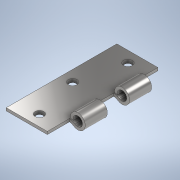
# Autodesk Inventor part: Hinge1
Saved by Autodesk Inventor 2021 (Build 250183000, 183)
## iProperties
Created: 2021-07-31
Part Number: Hinge1
Material: Stainless Steel
Document SubType Name: Modeling
Designer: Shammy Haider
Density: 8 g/cm^3
Appearance: Semi-Polished
Author: Shammy Haider
Autodesk Inventor part; units mm, degrees
ref_plane "YZ Plane" through (0, 0, 0) normal (1, 0, 0) x (0, 1, 0)
ref_plane "XZ Plane" through (0, 0, 0) normal (0, 1, 0) x (-1, 0, 0)
ref_plane "XY Plane" through (0, 0, 0) normal (0, 0, 1) x (1, 0, 0)
sketch "Sketch1" plane through (0, 0, 0) normal (0, 0, 1) x (1, 0, 0)
  line L0 (-44.6809, 2.5) -> (-7.5647, 2.5)
  line L1 (-44.6809, 0) -> (-44.6809, 2.5)
  line L2 (0, 0) -> (0, 19.2246)
  arc A0 (-3.8253, -1.3563) -> (-6.7141, 3.5099) centre (0, 4.2052) ccw
  arc A1 (-2.5687, 0.8193) -> (-4.0285, 2.8511) centre (0, 4.2052) ccw
  arc A2 (-2.5687, 0.8193) -> (-7.5647, 2.5) centre (-7.5647, -5.7659) ccw
  line L3 (-4.0285, 2.8511) -> (-6.7141, 3.5099)
  arc A3 (-3.8253, -1.3563) -> (-8.1904, 0) centre (-8.1904, -7.7027) ccw
  line L4 (-8.1904, 0) -> (-44.6809, 0)
  line L5 (-36.0171, 0) -> (-5.5909, 0)
  line L6 (-5.2801, 0) -> (0, 0)
  point P0 (0, 10.9552)
  point P1 (0, 8.4552)
  dimension "d1" = 2.5
  dimension "d2" = 2.5
  dimension "d3" = 8.5
  constraints: 14 end point, 8 point on circle, 4 centre point, 4 tangent, 3 horizontal, 2 collinear, 2 perpendicular, 2 point on line, 1 coincident, 1 parallel
  measures "d1" distance of L1.start L0.start
  measures "d2" radial gap between concentric circles of A1 A0
  measures "d3" diameter of A1
extrude "Extrusion1" add sketch "Sketch1" along normal mid plane 100 contours L0 A2 A1 L2 A0 A3 L4 L1 | A1 L3 A0 L2
sketch "Sketch2" plane through (-44.6809, 2.5, 50) normal (0, 1, 0) x (1, 0, 0)
  circle A0 centre (20, 90) radius 4
  circle A1 centre (10, 50) radius 4
  circle A2 centre (20, 10) radius 4
  line L0 (0, 100) -> (37.1161, 100) projected
  line L1 (0, 100) -> (0, 0) projected
  line L2 (37.1161, 0) -> (0, 0) projected
  point P0 (44.6809, 50)
  dimension "d6" = 8
  dimension "d7" = 8
  dimension "d8" = 8
  dimension "d9" = 10
  dimension "d10" = 20
  dimension "d11" = 20
  dimension "d12" = 10
  dimension "d13" = 10
  dimension "d14" = 50
  constraints: 3 centre point
  measures "d6" diameter of A0
  measures "d7" diameter of A1
  measures "d8" diameter of A2
  measures "d9" distance from line of L0 A0.centre
  measures "d10" distance from line of L1 A0.centre
  measures "d11" distance from line of L1 A2.centre
  measures "d12" distance from line of L2 A2.centre
  measures "d13" distance from line of L1 A1.centre
  measures "d14" distance from line of L2 A1.centre
extrude "Extrusion2" cut sketch "Sketch2" against normal up to next draft -20
sketch "Sketch3" plane through (-44.6809, 2.5, 50) normal (0, 1, 0) x (1, 0, 0)
  line L0 (37.1161, 0) -> (37.1161, 100) projected
  line L1 (37.1161, 100) -> (67.1161, 100)
  line L2 (67.1161, 100) -> (67.1161, 80)
  line L3 (67.1161, 80) -> (37.1161, 80)
  line L4 (37.1161, 80) -> (37.1161, 100)
  line L5 (37.1161, 60) -> (67.1161, 60)
  line L6 (67.1161, 60) -> (67.1161, 40)
  line L7 (67.1161, 40) -> (37.1161, 40)
  line L8 (37.1161, 40) -> (37.1161, 60)
  line L9 (37.1161, 0) -> (0, 0) projected
  line L10 (37.1161, 0) -> (70.6977, 0)
  line L11 (70.6977, 0) -> (70.6977, 20)
  line L12 (70.6977, 20) -> (37.1161, 20)
  line L13 (37.1161, 20) -> (37.1161, 0)
  point P0 (44.6809, 50)
  point P1 (37.1161, 20)
  dimension "d17" = 20
  dimension "d18" = 30
  dimension "d19" = 20
  dimension "d20" = 20
  dimension "d21" = 20
  constraints: 24 end point, 6 parallel, 3 horizontal, 3 perpendicular, 1 point on line
  measures "d17" distance of L1.end L2.end
  measures "d18" distance of L0.end L1.end
  measures "d19" distance of L5.end L6.end
  measures "d20" distance of L10.end L11.end
  measures "d21" distance between parallel lines of L5 L3
extrude "Extrusion3" cut sketch "Sketch3" against normal mid plane 100
body "Solid1"
